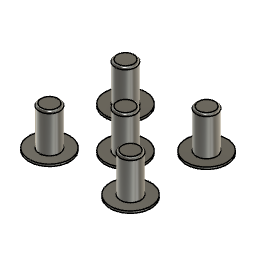
boutons (Autodesk Fusion 360 design; units mm, degrees)
Autodesk Fusion 360 part; units mm, degrees
sketch "Esquisse1" plane through (0, 0, 0) normal (0, 0, 1) x (1, 0, 0)
  circle A0 centre (0, 0) radius 2
  circle A1 centre (0, 0) radius 4
  dimension "d1" = 4
  dimension "d2" = 2
  constraint coincident A0.centre A1.centre
  measures "d1" diameter of A0
  measures "d2" distance of A0
extrude "Extrusion1" add sketch "Esquisse1" along normal blind 0.4 makes body 1
extrude "Extrusion2" add sketch "Esquisse1" along normal blind 8 contours A0 bodies 1
fillet "Congé1" radius 0.4 1 edges at (-1.8647, -0.7232, 8) on bodies 1
copy_body "Copier/Coller des corps1" bodies 1 makes body 2
move_body "Déplacer1" bodies 2 to x (1, 0, 0) y (0, 1, 0) z (0, 0, 1) at (9, 0, 0)
copy_body "Copier/Coller des corps2" bodies 1 makes body 3
move_body "Déplacer2" bodies 3 to x (1, 0, 0) y (0, 1, 0) z (0, 0, 1) at (0, 9, 0)
copy_body "Copier/Coller des corps3" bodies 1 makes body 4
move_body "Déplacer3" bodies 4 to x (1, 0, 0) y (0, 1, 0) z (0, 0, 1) at (9, 11, 0)
move_body "Déplacer4" bodies 3 to x (1, 0, 0) y (0, 1, 0) z (0, 0, 1) at (0, 2, 0)
move_body "Déplacer5" bodies 2 4 to x (1, 0, 0) y (0, 1, 0) z (0, 0, 1) at (5, 0, 0)
copy_body "Copier/Coller des corps4" bodies 1 makes body 5
move_body "Déplacer6" bodies 5 to x (1, 0, 0) y (0, 1, 0) z (0, 0, 1) at (7, 6, 0)
move_body "Déplacer7" bodies 3 4 to x (1, 0, 0) y (0, 1, 0) z (0, 0, 1) at (0, 2, 0)
move_body "Déplacer8" bodies 4 2 to x (1, 0, 0) y (0, 1, 0) z (0, 0, 1) at (2, 0, 0)
move_body "Déplacer9" bodies 3 4 to x (1, 0, 0) y (0, 1, 0) z (0, 0, 1) at (0, 2, 0)
move_body "Déplacer10" bodies 5 to x (1, 0, 0) y (0, 1, 0) z (0, 0, 1) at (1, 1, 0)
